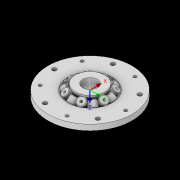
# Autodesk Inventor part: OuterBearing_TBS
Saved by Autodesk Inventor 2022.2 (Build 262287010, 287A)
## iProperties
Created: 2022-05-21
Part Number: OuterBearing_TBS
Material: Generic
Document SubType Name: Modeling
Designer: Árni Þór Þorgeirsson
Density: 1 g/cm^3
Appearance: Default
Author: Árni Þór Þorgeirsson
Autodesk Inventor part; units mm, degrees
ref_plane "YZ Plane" through (0, 0, 0) normal (1, 0, 0) x (0, 1, 0)
ref_plane "XZ Plane" through (0, 0, 0) normal (0, 1, 0) x (-1, 0, 0)
sketch "Sketch1" plane through (0, 0, 0) normal (0, 0, 1) x (1, 0, 0)
  circle A0 centre (0, 0) radius 15.781563 construction
  line L0 (0, 0) -> (15.781563, 0)
  line L1 (0, 0) -> (15.781563, 4.025)
  line L2 (15.781563, 0) -> (15.781563, 4.025)
  circle A1 centre (0, 0) radius 40
  dimension "d56" = 15.78156
  dimension "d57" = 4.025
  dimension "d400" = 40
  dimension "d495" = 2.5
  dimension "d496" = 8
  dimension "d531" = 5.5
  dimension "d532" = 5.5
  dimension "d533" = 5.5
  dimension "d537" = 24.5
  dimension "d538" = 3
  dimension "d543" = 5.5
  dimension "d549" = 3
  dimension "d550" = 3
  dimension "d567" = 5.5
  dimension "d568" = 5.5
  constraints: 1 other
sketch "Sketch7" plane through (0, 0, 0) normal (0, 1, 0) x (-1, 0, 0)
  line L0 (0, 0) -> (0, 18.336628)
  line L1 (0, 0) -> (-15.781563, 0) construction
  line L2 (0, 18.336628) -> (-15.781563, 0) construction
  line L3 (0, 18.336628) -> (-21.121605, 0) construction
  line L4 (0, 18.336628) -> (-15.005003, -5.310101) construction
  line L5 (0, 0) -> (0, -18.336628)
  line L6 (0, -18.336628) -> (-15.781563, 0) construction
  line L7 (0, -18.336628) -> (-21.121605, 0) construction
  line L8 (0, -18.336628) -> (-15.005003, 5.310101) construction
  line L9 (-15.005003, 5.310101) -> (-21.121605, 0) construction
  line L10 (-11.635485, 0) -> (-20.775221, -7.934622) construction
  line L11 (-11.635485, 0) -> (-19.424414, 6.761925) construction
  line L12 (0, -42.003954) -> (0, 123.667326)
  line L13 (-40, -5.99191) -> (-40, 6.008042)
  line L14 (106.88681, 0) -> (-116.32086, 0)
  line L15 (-18.463148, 2.307928) -> (-13.099977, -2.307928) construction
  line L16 (-13.099977, 2.307928) -> (-18.463148, -2.307928) construction
  line L17 (-26.151002, -15.930308) -> (-40.378296, -15.930308) construction
  line L18 (-40.378296, -15.930308) -> (-40.378296, -12.753867) construction
  line L19 (-40.378296, -12.753867) -> (-26.151002, -12.753867) construction
  line L20 (-26.151002, -12.753867) -> (-26.151002, -15.930308) construction
  point P0 (-40, 0)
  dimension "Roller_Side_difference" = 0.491
  dimension "d90" = 18.33663
  dimension "d201" = 40
  dimension "d343" = 98.5656
  dimension "d344" = 98.0745
  dimension "d367" = 8.1
  constraints: 28 end point, 9 point on line, 3 midpoint, 3 vertical, 2 horizontal, 2 parallel, 2 perpendicular, 1 collinear, 1 symmetric about line, 2 other
  measures "d90" distance of L0.start L0.end
  measures "d201" distance between parallel lines of L5 L13
  measures "d343" angle of L10 L8
  measures "d344" angle of L7 L10
  measures "d367" distance of L3.end L8.end
sketch "Roller1" plane through (0, 0, 0) normal (0, 1, 0) x (-1, 0, 0)
  line L0 (0, 18.336628) -> (-15.005003, -5.310101) construction
  line L1 (0, 18.336628) -> (-21.121605, 0) construction
  line L2 (-11.635485, 0) -> (-19.424414, 6.761925) construction
  line L3 (0, -18.336628) -> (-21.121605, 0) construction
  line L4 (-11.708759, -0.068814) -> (-14.969911, -5.208139)
  line L5 (-14.969911, -5.208139) -> (-21.026268, 0.04966)
  line L6 (-21.026268, 0.04966) -> (-16.435747, 4.0349)
  line L7 (-16.435747, 4.0349) -> (-11.708759, -0.068814)
  line L8 (-13.297441, 1.310393) -> (-17.243172, -3.234618)
  line L9 (-17.99809, -2.57924) -> (-14.052358, 1.965772)
  point P0 (0, 0)
  dimension "d345" = 0.025
  dimension "d346" = 0.025
  dimension "d347" = 0.1
  dimension "d348" = 0.1
  dimension "d349" = 98.0745
  dimension "d350" = 98.5656
  dimension "d617" = 0.99971
  constraints: 12 end point, 4 parallel, 3 point on line, 1 midpoint, 1 perpendicular
  measures "d345" distance between parallel lines of L0 L4
  measures "d346" distance between parallel lines of L1 L6
  measures "d347" distance between parallel lines of L3 L5
  measures "d348" distance between parallel lines of L2 L7
  measures "d349" angle of L6 L7
  measures "d350" angle of L4 L7
  measures "d617" distance between parallel lines of L9 L8
sketch "Roller2" plane through (0, 0, 0) normal (0, 1, 0) x (-1, 0, 0)
  line L0 (0, -18.336628) -> (-15.005003, 5.310101) construction
  line L1 (-11.635485, 0) -> (-20.775221, -7.934622) construction
  line L2 (0, -18.336628) -> (-21.121605, 0) construction
  line L3 (0, 18.336628) -> (-21.121605, 0) construction
  line L4 (-15.010548, 5.27218) -> (-11.668122, 0.004773)
  line L5 (-11.668122, 0.004773) -> (-16.378545, -4.08456)
  line L6 (-16.378545, -4.08456) -> (-21.08347, 0)
  line L7 (-21.08347, 0) -> (-15.010548, 5.27218)
  line L8 (-18.047009, 2.63609) -> (-14.002942, -2.022192)
  line L9 (-17.291873, 3.291658) -> (-13.247806, -1.366623)
  point P0 (0, 0)
  dimension "d351" = 0.025
  dimension "d352" = 0.025
  dimension "d354" = 0.025
  dimension "d355" = 98.5656
  dimension "d356" = 98.0745
  dimension "d370" = 0.025
  dimension "d371" = 1
  constraints: 12 end point, 5 parallel, 3 point on line, 1 midpoint, 1 perpendicular
  measures "d351" distance between parallel lines of L0 L4
  measures "d352" distance between parallel lines of L2 L6
  measures "d354" distance between parallel lines of L1 L5
  measures "d355" angle of L5 L4
  measures "d356" angle of L6 L5
  measures "d370" distance from line of L3 L8.start
  measures "d371" distance between parallel lines of L9 L8
sketch "Sketch22" plane through (0, 0, 0) normal (0, 1, 0) x (-1, 0, 0)
  line L0 (-31.75595, 8.021531) -> (-17.528657, 8.021531) construction
  line L1 (-17.528657, 8.021531) -> (-17.528657, 4.84509) construction
  line L2 (-17.528657, 4.84509) -> (-31.75595, 4.84509) construction
  line L3 (-31.75595, 4.84509) -> (-31.75595, 8.021531) construction
  point P0 (0, 0)
  dimension "Roller_Side_difference" = 0.491
  constraints: 2 other
sketch "Sketch2" plane through (0, 0, 0) normal (0, 1, 0) x (-1, 0, 0)
  line L0 (0, 0) -> (0, 15.781563) construction
  line L1 (0, 0) -> (-15.781563, 0)
  line L2 (0, 0) -> (0, -15.781563)
  line L3 (0, -15.781563) -> (-15.781563, 0) construction
  line L4 (0, 15.781563) -> (-15.781563, 0) construction
  line L5 (-84.43405, 62.544519) -> (0, 15.781563) construction
  line L6 (-35.133225, 16.810121) -> (0, 15.781563) construction
  line L7 (-35.133225, 16.810121) -> (0, -15.781563) construction
  line L8 (-48.838086, 17.211344) -> (0, -15.781563) construction
  point P0 (-18.693155, -2.911593)
  constraints: 16 end point, 3 point on line, 1 perpendicular, 1 symmetric about line, 1 vertical
sketch "Sketch23" plane through (0, 0, 0) normal (0, 1, 0) x (-1, 0, 0)
  line L0 (0, -18.336628) -> (-15.005003, 5.310101) construction
  line L1 (0, -18.336628) -> (-21.121605, 0) construction
  line L2 (0, 18.336628) -> (-15.005003, -5.310101) construction
  line L3 (-15.005003, 5.310101) -> (-21.121605, 0) construction
  line L4 (0, 18.336628) -> (-21.121605, 0) construction
  line L5 (-15.005003, 5.310101) -> (-15.005003, -5.310101) construction
  line L6 (106.88681, 0) -> (-116.32086, 0)
  line L7 (-14.023571, 3.810101) -> (-11.639874, 0.053578)
  line L8 (-11.639874, -0.053578) -> (-14.023571, -3.810101)
  line L9 (-16.770958, 3.810101) -> (-21.072757, 0.075514)
  line L10 (-21.072757, -0.075514) -> (-16.770958, -3.810101)
  arc A0 (-21.072757, 0.075514) -> (-21.072757, -0.075514) centre (-21.0072, 0) ccw
  arc A1 (-11.639874, -0.053578) -> (-11.639874, 0.053578) centre (-11.72431, 0) ccw
  line L11 (-14.023571, 3.810101) -> (-14.023571, 5.310101)
  line L12 (-14.023571, 5.310101) -> (-7, 5.310101)
  line L13 (-7, 5.310101) -> (-7, -5.310101)
  line L14 (-7, -5.310101) -> (-14.023571, -5.310101)
  line L15 (-14.023571, -5.310101) -> (-14.023571, -3.810101)
  line L16 (-16.770958, 3.810101) -> (-16.770958, 5.310101)
  line L17 (-16.770958, 5.310101) -> (-40, 5.310101)
  line L18 (-40, 5.310101) -> (-40, -5.310101)
  line L19 (-16.770958, -3.810101) -> (-16.770958, -5.310101)
  line L20 (-16.770958, -5.310101) -> (-40, -5.310101)
  line L21 (-15.005003, 5.310101) -> (-15.005003, 5.310101)
  line L22 (-15.005003, -5.310101) -> (-15.005003, -5.310101)
  line L23 (0, -42.003954) -> (0, 123.667326)
  line L24 (-21.15974, 0) -> (-40, 0)
  point P0 (0, 0)
  point P1 (-11.605876, 0)
  point P2 (-21.1072, 0)
  point P3 (-40, 0)
  dimension "d378" = 90
  dimension "d379" = 0.1
  dimension "d380" = 0.025
  dimension "d381" = 0.025
  dimension "d382" = 0.025
  dimension "d383" = 0.025
  dimension "d384" = 10.6202
  dimension "d385" = 0
  dimension "d386" = 0
  dimension "d391" = 7
  dimension "d392" = 40
  dimension "d393" = 1.5
  dimension "d394" = 1.5
  dimension "d395" = 1.5
  dimension "d396" = 1.5
  constraints: 36 end point, 10 point on line, 9 vertical, 4 horizontal, 4 parallel, 4 point on circle, 4 tangent, 2 centre point, 1 equal radius, 1 midpoint
  measures "d378" angle of L6 L5
  measures "d379" radius of A0
  measures "d380" distance between parallel lines of L9 L4
  measures "d381" distance between parallel lines of L10 L1
  measures "d382" distance between parallel lines of L0 L7
  measures "d383" distance between parallel lines of L2 L8
  measures "d384" distance of L0.end L2.end
  measures "d385" distance of L2.end L22.end
  measures "d386" distance of L0.end L21.end
  measures "d391" distance between parallel lines of L23 L13
  measures "d392" distance between parallel lines of L18 L23
  measures "d393" distance of L9.start L16.end
  measures "d394" distance of L7.start L11.end
  measures "d395" distance of L14.end L8.end
  measures "d396" distance of L10.end L19.end
revolve "RevRoller1" add sketch "Roller1" angle 360 about axis through (17.99809, 0, -2.57924) along (-0.6555681, 0, 0.7551361) contours L4 L5 L8 L7
fillet "Fillet1" radius 0.5 2 edges at (16.396, 0, 4.0004) (21.0263, 0, 0.0497)
sketch "Sketch48" plane through (14.052358, 0, 1.965772) normal (-0.6555681, 0, 0.7551361) x (0.7551361, 0, 0.6555681)
  line L0 (-2.5, 0.25) -> (2.5, 0.25)
  line L1 (2.5, 0.25) -> (2.5, -0.25)
  line L2 (2.5, -0.25) -> (-2.5, -0.25)
  line L3 (-2.5, -0.25) -> (-2.5, 0.25)
  line L4 (-2.5, 0.25) -> (2.5, -0.25) construction
  line L5 (2.5, 0.25) -> (-2.5, -0.25) construction
  line L6 (-0.25, -2.5) -> (0.25, -2.5)
  line L7 (0.25, -2.5) -> (0.25, 2.5)
  line L8 (0.25, 2.5) -> (-0.25, 2.5)
  line L9 (-0.25, 2.5) -> (-0.25, -2.5)
  line L10 (-0.25, -2.5) -> (0.25, 2.5) construction
  line L11 (0.25, -2.5) -> (-0.25, 2.5) construction
  point P0 (-11.90014, 0)
  point P1 (0, 0)
  point P2 (-0.25, 0.25)
  point P3 (-0.25, -0.25)
  point P4 (0.25, -0.25)
  point P5 (0.25, 0.25)
  dimension "d621" = 5
  dimension "d622" = 0.5
  dimension "d623" = 0.5
  dimension "d624" = 5
  constraints: 24 end point, 4 midpoint, 4 parallel, 2 horizontal, 2 perpendicular
  measures "d621" distance of L1.end L2.end
  measures "d622" distance of L0.end L1.end
  measures "d623" distance of L8.end L7.end
  measures "d624" distance of L7.end L6.end
extrude "Extrusion39" cut sketch "Sketch48" against normal blind 0.2
pattern_circular "Circular Pattern13" count 7 over 360 about axis through (0, 0, -10) along (0, 0, 1) of "RevRoller1", "Fillet1"
move or copy body "Move Body7" bodies to move or copy 1 copy no rotation origin (0, 0, 0) rotation axis (0, 0, 1) rotation angle 25.714286
revolve "Revolution13" add sketch "Roller2" angle 360 about axis through (18.047009, 0, 2.63609) along (-0.6555681, 0, -0.7551361) contours L4 L5 L9 L7
fillet "Fillet3" radius 0.5 2 edges at (21.0835, 0, 0) (16.3378, 0, -4.0492)
pattern_circular "Circular Pattern14" count 7 over 360 about axis through (0, 0, -10) along (0, 0, 1) of "Revolution13", "Fillet3"
move or copy body "Move Body6" bodies to move or copy 1 copy no rotation origin (0, 0, 0) rotation axis (0, 0, 1) rotation angle 25.714286
revolve "Revolution14" add sketch "Sketch23" angle 360 about axis through (0, 0, -10) along (0, 0, 1) contours L13 L14 L15 L8 A1 L6 | L6 A1 L7 L11 L12 L13
revolve "OuterRim_Top2" [suppressed]
revolve "OuterRim_Bottom2" add sketch "Sketch23" angle 360 about axis through (0, 0, -10) along (0, 0, 1) contours L6 L18 L17 L16 L9 A0
ref_plane "Work Plane8" through (0, 0, 20) normal (0, 0, 1) x (1, 0, 0)
sketch "Sketch49" plane through (0, 0, 20) normal (0, 0, 1) x (1, 0, 0)
  circle A0 centre (0, 0) radius 40
  circle A1 centre (0, 0) radius 16.770958
  circle A2 centre (0, 0) radius 14.023571
  circle A3 centre (0, 0) radius 7
  circle A4 centre (0, 0) radius 34
  circle A5 centre (0, 0) radius 24.25
  point P0 (0, 34)
  point P1 (0, 24.25)
  point P2 (-19.984699, 27.506578)
  dimension "d629" = 34
  dimension "d630" = 48.5
  dimension "d649" = 36
  constraints: 2 coincident, 2 vertical alignment, 6 other
sketch "Sketch50" plane through (0, 0, 5.310101) normal (0, 0, 1) x (1, 0, 0)
  point P0 (0, 0)
  point P1 (0, 34)
sketch "Sketch51" plane through (0, 0, -5.520307) normal (0, 0, -1) x (-1, 0, 0)
  circle A0 centre (0, 0) radius 60
  circle A1 centre (0, 54) radius 2.75
  circle A2 centre (0, 54) radius 1.5
  circle A3 centre (-31.740404, 43.686918) radius 3.5
  circle A4 centre (-31.740404, 43.686918) radius 2
  dimension "d633" = 36
  dimension "d635" = 5.5
  dimension "d636" = 3
  dimension "d637" = 7
  dimension "d638" = 4
  constraints: 4 centre point, 4 coincident, 2 other
  measures "d635" diameter of A1
  measures "d636" diameter of A2
  measures "d637" diameter of A3
  measures "d638" diameter of A4
extrude "Extrusion40" [suppressed]
extrude "Extrusion41" [suppressed]
extrude "Extrusion42" [suppressed]
extrude "Extrusion43" [suppressed]
sketch "Sketch52" plane through (0, 0, 5.310101) normal (0, 0, 1) x (1, 0, 0)
  circle A0 centre (0, 34) radius 1.5
  circle A1 centre (-19.984699, 27.506578) radius 2
  line L0 (2.75, 32.412287) -> (0, 30.824574)
  line L1 (0, 30.824574) -> (-2.75, 32.412287)
  line L2 (-2.75, 32.412287) -> (-2.75, 35.587713)
  line L3 (-2.75, 35.587713) -> (0, 37.175426)
  line L4 (0, 37.175426) -> (2.75, 35.587713)
  line L5 (2.75, 35.587713) -> (2.75, 32.412287)
  circle A2 centre (0, 0) radius 40
  line L6 (-18.693136, 30.407474) -> (-16.826667, 27.8385)
  line L7 (-15.965386, 27.929025) -> (-17.609193, 24.236975)
  line L8 (-17.609193, 24.236975) -> (-21.628505, 23.814528)
  line L9 (-21.628505, 23.814528) -> (-24.004011, 27.084131)
  line L10 (-24.004011, 27.084131) -> (-22.360204, 30.776181)
  line L11 (-22.360204, 30.776181) -> (-18.340892, 31.198628)
  line L12 (-18.340892, 31.198628) -> (-15.965386, 27.929025)
  dimension "d651" = 3
  dimension "d652" = 4
  dimension "d655" = 36
  dimension "d657" = 7
  dimension "d658" = 5.5
  constraints: 26 end point, 4 coincident, 2 centre point, 1 parallel, 30 other
  measures "d651" diameter of A0
  measures "d652" diameter of A1
  measures "d657" distance between parallel lines of L12 L9
  measures "d658" distance between parallel lines of L5 L2
extrude "Extrusion44" cut sketch "Sketch52" against normal blind 5.310101 contours A0
extrude "Extrusion45" cut sketch "Sketch52" against normal blind 2.020203 contours A0 | L0 L1 L2 L3 L4 L5
extrude "Extrusion46" cut sketch "Sketch52" against normal blind 5.310101 contours A1
extrude "Extrusion47" cut sketch "Sketch52" against normal blind 2.620203 contours A1 | L7 L8 L9 L10 L11 L12
pattern_circular "Circular Pattern32" [suppressed]
pattern_circular "Circular Pattern33" count 5 over 360 about axis through (0, 0, 4.560101) along (0, 0, 1) of "Extrusion44", "Extrusion45", "Extrusion46", "Extrusion47"
sketch "Sketch57" plane through (0, 0, -5.310101) normal (0, 0, -1) x (-1, 0, 0)
  line L0 (-3.175, 27.425) -> (3.175, 27.425)
  line L1 (3.175, 27.425) -> (3.175, 21.075)
  line L2 (3.175, 21.075) -> (-3.175, 21.075)
  line L3 (-3.175, 21.075) -> (-3.175, 27.425)
  line L4 (-3.175, 27.425) -> (3.175, 21.075) construction
  line L5 (3.175, 27.425) -> (-3.175, 21.075) construction
  ellipse E0 centre (0, 24.25) end of major axis (6.4, 24.25) minor radius 5.45
  point P0 (0, 0)
  dimension "d694" = 6.35
  dimension "d695" = 6.35
  dimension "d696" = 6.4
  dimension "d697" = 5.45
  constraints: 1 coincident, 1 vertical alignment, 2 other
  measures "d694" distance of L1.end L2.end
  measures "d695" distance of L0.end L1.end
sketch "Sketch40" plane through (0, 0, -5.230953) normal (0, 0, -1) x (-1, 0, 0)
  circle A0 centre (53.5, 0) radius 2.75 projected
  circle A1 centre (0, 0) radius 53.5 projected
  point P0 (53.429322, 2.749092)
  point P1 (53.429322, -2.749092)
  dimension "d585" = 8
  dimension "d587" = 1.75
  dimension "d589" = 3
  dimension "d592" = 2
  dimension "d593" = 12
  dimension "d594" = 12
  dimension "d611" = 360
  constraints: 18 point on circle, 10 centre point, 8 end point, 2 midpoint, 1 horizontal alignment, 1 vertical, 29 other
  measures "d589" diameter of A1
equation "\"Roller_Side_difference\" = 0.491096deg"
equation "\"Cycloid_Top_Plate_Fasner_Inner\" = 61.25"
equation "\"Cycloid_Top_Plate_Fasner_Outer\" = 85.75"
equation "\"Roller_Hole_Radius\" = 1"
equation "\"Distance_To_Bearing\" = 24.19276"
equation "\"d514\" = 0.2"
equation "\"Machine_Screw_4mm_Head_Dept\" = 4"
equation "\"Machine_Screw_4mm_Head_Diameter\" = 7"
equation "\"Machine_Screw_4mm_HexNut_Thickness\" = 3"
equation "\"Machine_Screw_4mm_HexNut_Width\" = 6.9"
equation "\"Machine_Screw_4mm_Length\" = 8"
equation "\"Fastner_4mm_Hex_Nut_Width\" = 7"
equation "\"Fastner_4mm_Screw_Diameter\" = 4"
equation "\"Fastner_4mm_Screw_Head_Diameter\" = 7"
equation "\"Fastner_4mm_Hex_Nut_Hole_Dept\" = 2.6202"
equation "\"Fastner_4mm_Screw_Head_Hole_Dept\" = 4"
body "Solid1"
body "Solid5"
